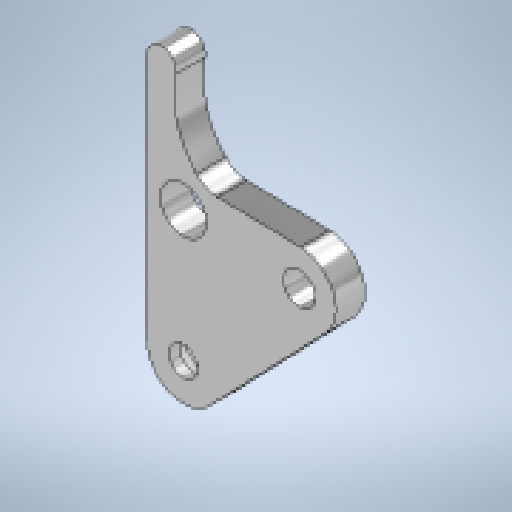
# Autodesk Inventor part: Lever
Saved by Autodesk Inventor 2023.2 (Build 272271000, 271)
## iProperties
Created: 2024-01-16
Part Number: Lever
Material: Aluminum 6061
Document SubType Name: Modeling
Designer: Nathan Cai
Mass: 3.70951 g
Surface Area: 13.9952 cm^2
Volume: 1.37389 cm^3
Density: 2.7 g/cm^3
Appearance: Aluminum - Flat
Lever_Offset: 0.625 in
Lever_Angle: 97.50 deg
Author: Nathan Cai
Autodesk Inventor part; units mm, degrees
ref_plane "YZ Plane" through (0, 0, 0) normal (1, 0, 0) x (0, 1, 0)
ref_plane "XZ Plane" through (0, 0, 0) normal (0, 1, 0) x (-1, 0, 0)
ref_plane "XY Plane" through (0, 0, 0) normal (0, 0, 1) x (1, 0, 0)
sketch "Sketch4" plane through (0, 0, 0) normal (0, 0, 1) x (1, 0, 0)
  circle A0 centre (0, 0) radius 2.5083
  circle A1 centre (0, 0) radius 3.9688
  line L0 (-3.9688, 0) -> (-3.9688, 12.7)
  arc A2 (-0.8259, 12.3821) -> (-3.9688, 12.7) centre (-2.3812, 12.7) ccw
  arc A3 (-0.8259, 12.3821) -> (2.5018, 3.0809) centre (8.5062, 10.475) ccw
  circle A4 centre (0, 0) radius 4.7625 construction
  circle A5 centre (15.7392, -2.0721) radius 6.35 construction
  circle A6 centre (15.7392, -2.0721) radius 3.9688
  circle A7 centre (15.7392, -2.0721) radius 1.7526
  line L1 (2.5018, 3.0809) -> (16.0883, 1.8813)
  circle A8 centre (-2.532, -12.445) radius 3.9688
  circle A9 centre (-2.532, -12.445) radius 1.5875
  line L2 (-6.421, -11.6538) -> (-3.8891, 0.7912)
  line L3 (17.6986, -5.5234) -> (-0.5726, -15.8964)
  line L4 (0, 0) -> (15.7392, -2.0721) construction
  line L5 (15.7392, -2.0721) -> (16.2572, 1.8627) construction
  line L6 (0, 4.7625) -> (0, 0) construction
  line L7 (-2.532, -12.445) -> (0, 0) construction
  line L8 (-2.532, -12.445) -> (-4.0876, -12.1285) construction
  circle A10 centre (-2.532, -12.445) radius 4.7625 construction
  arc A11 (15.0853, -5.9866) -> (1.1645, -13.8898) centre (12.993, -18.5131) ccw
  point P0 (3.9688, 0)
  point P1 (2.0561, -3.3946)
  dimension "d54" = 9.525
  dimension "d62" = 3.175
  dimension "d44" = 5.0165
  dimension "d45" = 7.9375
  dimension "d51" = 12.7
  dimension "d52" = 3.175
  dimension "d53" = 9.525
  dimension "d56" = 12.7
  dimension "d57" = 7.9375
  dimension "d58" = 3.5052
  dimension "d61" = 7.9375
  dimension "Lever_Offset" = 15.875
  dimension "Lever_Angle" = 97.5
  dimension "d72" = 191.5
  dimension "d73" = 12.7
  dimension "d74" = 9.525
  dimension "d75" = 25.4
  constraints: 18 end point, 18 point on circle, 11 tangent, 10 centre point, 7 coincident, 2 perpendicular, 2 vertical, 1 vertical alignment, 5 other
  measures "d44" diameter of A0
  measures "d45" diameter of A1
  measures "d51" distance of L0.start L0.end
  measures "d52" diameter of A2
  measures "d53" radius of A3
  measures "d56" diameter of A5
  measures "d57" diameter of A6
  measures "d58" diameter of A7
  measures "d61" diameter of A8
  measures "Lever_Offset" distance from line of point (0, 0) L5
  measures "Lever_Angle" angle of L6 L4
  measures "d73" distance from line of point (0, 0) L8
  measures "d74" diameter of A10
  measures "d75" diameter of A11
extrude "Extrusion3" add sketch "Sketch4" along normal blind 7.9375 contours A1 | A1 L1 A6 A11 A8 L2 L0 | A1 L2 L0 A2 A3 | L0 L2 A1 | A6 | A8
fillet "Fillet5" radius 3.175 2 edges at (2.5018, 3.0809, 3.9688) (-3.9688, 0.3996, 3.9688)
sketch "Sketch5" plane through (0, 0, 7.9375) normal (0, 0, 1) x (1, 0, 0)
  arc A0 (15.0853, -5.9866) -> (16.0883, 1.8813) centre (15.7392, -2.0721) ccw projected
  arc A1 (-0.8259, 12.3821) -> (1.5343, 3.9852) centre (8.5062, 10.475) ccw projected
  arc A2 (-0.8259, 12.3821) -> (-3.9688, 12.7) centre (-2.3812, 12.7) ccw projected
  arc A3 (-6.421, -11.6538) -> (1.1645, -13.8898) centre (-2.532, -12.445) ccw projected
  circle A4 centre (-2.532, -12.445) radius 6.35
  circle A5 centre (0, 0) radius 3.9688
  circle A6 centre (15.7392, -2.0721) radius 6.4439
  line L0 (-4.0325, 0.0863) -> (-6.421, -11.6538) projected
  line L1 (16.0883, 1.8813) -> (3.579, 2.9858) projected
  arc A7 (1.5343, 3.9852) -> (3.579, 2.9858) centre (3.8582, 6.1485) ccw projected
  circle A8 centre (0, 0) radius 2.5083 projected
  line L2 (-3.9688, 12.7) -> (-3.9688, 0.7193) projected
  arc A9 (-4.0325, 0.0863) -> (-3.9688, 0.7193) centre (-7.1437, 0.7193) ccw projected
  arc A10 (15.0853, -5.9866) -> (1.1645, -13.8898) centre (12.993, -18.5131) ccw projected
  point P0 (-3.9688, 0)
  point P1 (15.0677, -4.2555)
  point P2 (12.7369, 2.861)
  point P3 (11.0312, 2.3278)
  point P4 (10.6542, -6.0303)
  dimension "d76" = 12.7
  constraints: 3 centre point, 2 coincident, 1 concentric
  measures "d76" diameter of A4
extrude "Extrusion4" cut sketch "Sketch5" against normal blind 4.7625 contours A10 A3 L0 A4 | A4 L0 A3 A10
chamfer "Chamfer2" distance 1.778 angle 49 1 edges at (-4.1195, -12.445, 0) measured on face at (8.6395, -2.6642, 0)
fillet "Fillet6" radius 6.35 2 edges at (-5.4328, -6.7963, 5.5563) (3.403, -10.1871, 5.5563)
body "Solid2"
